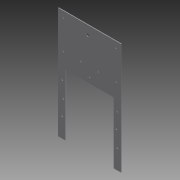
# Autodesk Inventor part: bottom plate
Saved by Autodesk Inventor 2011 SP1 (Build 150282100, 282)
## iProperties
Created: 2012-01-20
Part Number: bottom plate
Document SubType Name: Modeling
Designer: Christopher
Density: 1 g/cm^3
Author: Christopher
Autodesk Inventor part; units mm, degrees
ref_plane "YZ Plane" through (0, 0, 0) normal (1, 0, 0) x (0, 1, 0)
ref_plane "XZ Plane" through (0, 0, 0) normal (0, 1, 0) x (-1, 0, 0)
ref_plane "XY Plane" through (0, 0, 0) normal (0, 0, 1) x (1, 0, 0)
sketch "Sketch1" plane through (0, 0, 0) normal (0, 0, 1) x (1, 0, 0)
  line L0 (333.7348, 101.6) -> (333.7348, 584.2)
  line L1 (92.4348, 101.6) -> (92.4348, 368.3)
  line L2 (92.4348, 368.3) -> (301.9848, 368.3)
  line L3 (301.9848, 368.3) -> (301.9848, 101.6)
  line L4 (301.9848, 101.6) -> (333.7348, 101.6)
  line L5 (92.4348, 101.6) -> (60.6848, 101.6)
  line L6 (60.6848, 101.6) -> (60.6848, 584.2)
  line L7 (60.6848, 584.2) -> (333.7348, 584.2)
  point P0 (0, 0)
  point P1 (197.2098, 254)
  point P2 (197.2098, 391.541)
  point P3 (78.0958, 322.7705)
  point P4 (78.0958, 185.2295)
  point P5 (197.2098, 116.459)
  point P6 (316.3238, 185.2295)
  point P7 (316.3238, 322.7705)
  point P8 (187.6848, 546.1)
  point P9 (311.5098, 254)
  point P10 (311.5098, 558.8)
  point P11 (311.5098, 431.8)
  point P12 (82.9098, 558.8)
  point P13 (82.9098, 431.8)
  point P14 (82.9098, 254)
  point P15 (235.3098, 431.8)
  point P16 (159.1098, 431.8)
  dimension "d1" = 482.6
  dimension "d4" = 137.541
  dimension "d7" = 360
  dimension "d9" = 31.75
  dimension "d21" = 31.75
  dimension "d23" = 114.3
  dimension "d24" = 38.1
  dimension "d33" = 273.05
  dimension "d34" = 146.05
  dimension "d35" = 25.4
  dimension "d36" = 25.4
  dimension "d39" = 177.8
  dimension "d40" = 177.8
  dimension "d48" = 22.225
  dimension "d49" = 22.225
  dimension "d51" = 76.2
  dimension "d52" = 76.2
  dimension "d53" = 76.2
  dimension "d54" = 209.55
  dimension "d55" = 266.7
  dimension "d56" = 104.775
  dimension "d57" = 152.4
  dimension "d58" = 152.4
  constraints: 16 end point, 4 vertical alignment, 3 perpendicular, 2 horizontal alignment, 1 collinear, 1 parallel, 7 other
  measures "d1" distance of L0.end L0.start
  measures "d4" distance of point (197.21, 391.541) point (197.21, 254)
  measures "d9" distance between parallel lines of L0 L3
  measures "d21" distance of L1.start L5.end
  measures "d23" distance from line of point (197.21, 254) L2
  measures "d24" distance from line of L7 point (187.685, 546.1)
  measures "d33" distance of L6.end L0.end
  measures "d34" distance from line of L0 point (187.685, 546.1)
  measures "d35" distance from line of L7 point (311.51, 558.8)
  measures "d36" distance from line of L7 point (82.91, 558.8)
  measures "d39" distance of point (311.51, 254) point (311.51, 431.8)
  measures "d40" distance of point (82.91, 431.8) point (82.91, 254)
  measures "d48" distance from line of L6 point (82.91, 431.8)
  measures "d49" distance from line of L0 point (311.51, 431.8)
  measures "d51" distance of point (235.31, 431.8) point (311.51, 431.8)
  measures "d52" distance of point (159.11, 431.8) point (235.31, 431.8)
  measures "d53" distance of point (82.91, 431.8) point (159.11, 431.8)
  measures "d54" distance of L1.end L2.end
  measures "d55" distance of L2.end L3.end
  measures "d56" distance from line of L1 point (197.21, 254)
  measures "d57" distance from line of L4 point (311.51, 254)
  measures "d58" distance from line of L5 point (82.91, 254)
extrude "Extrusion1" add sketch "Sketch1" against normal blind 3.175
hole "Hole1" at (197.2098, 254, 0) at (197.2098, 391.541, 0) at (78.0958, 322.7705, 0) at (78.0958, 185.2295, 0) at (197.2098, 116.459, 0) at (316.3238, 185.2295, 0) at (316.3238, 322.7705, 0) direction (0, 0, -1) diameter 6.35 depth 25.4 tip angle 118
hole "Hole2" at (187.6848, 546.1, 0) direction (0, 0, -1) diameter 12.7 depth 25.4 tip angle 118
hole "Hole3" at (311.5098, 254, 0) at (311.5098, 558.8, 0) at (311.5098, 431.8, 0) at (82.9098, 558.8, 0) at (82.9098, 431.8, 0) at (82.9098, 254, 0) at (159.1098, 431.8, 0) at (235.3098, 431.8, 0) direction (0, 0, -1) diameter 6.35 depth 25.4 tip angle 118
body "Solid1"
